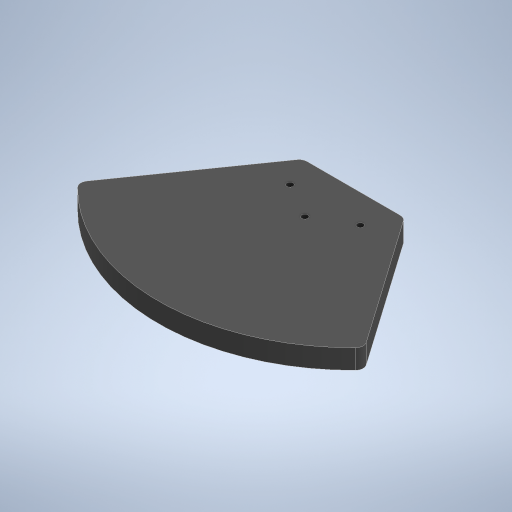
# Autodesk Inventor part: toe_sole_front
Saved by Autodesk Inventor 2024.1 (Build 281209000, 209)
## iProperties
Created: 2024-02-12
Part Number: toe_sole_front
Material: 一般
Document SubType Name: Modeling
Designer: hibik
Density: 1 g/cm^3
Appearance: 既定
Author: hibik
Autodesk Inventor part; units mm, degrees
ref_plane "YZ Plane" through (0, 0, 0) normal (1, 0, 0) x (0, 1, 0)
ref_plane "XZ Plane" through (0, 0, 0) normal (0, 1, 0) x (-1, 0, 0)
ref_plane "XY Plane" through (0, 0, 0) normal (0, 0, 1) x (1, 0, 0)
sketch "スケッチ1" plane through (0, 0, 0) normal (0, 1, 0) x (-1, 0, 0)
  line L0 (26, 0) -> (0, 0)
  line L1 (0, 0) -> (0, -15)
  line L2 (0, -15) -> (26, -15)
  line L3 (26, -15) -> (26, 0)
  line L4 (49.744, 13.9099) -> (26, -20)
  line L5 (26, -20) -> (0, -20)
  line L6 (0, -20) -> (-23.744, 13.9099)
  arc A0 (49.744, 13.9099) -> (-23.744, 13.9099) centre (13, -20) ccw
  line L7 (0, 0) -> (26, -15)
  line L8 (0, -15) -> (26, 0)
  line L9 (4, -2.3077) -> (22, -2.3077)
  line L10 (22, -2.3077) -> (22, -12.6923)
  line L11 (22, -12.6923) -> (4, -12.6923)
  line L12 (4, -12.6923) -> (4, -2.3077)
  circle A1 centre (4, -2.3077) radius 0.8
  circle A2 centre (4, -12.6923) radius 0.8
  circle A3 centre (22, -2.3077) radius 0.8
  circle A4 centre (22, -12.6923) radius 0.8
  circle A5 centre (13, -7.5) radius 0.8
  point P0 (22.6929, -13.0921)
  point P1 (21.2, -12.6923)
  dimension "d0" = 26
  dimension "d1" = 15
  dimension "d4" = 35
  dimension "d5" = 35
  dimension "d6" = 5
  dimension "d7" = 50
  dimension "d23" = 4
  dimension "d24" = 1.6
  dimension "d25" = 1.6
  dimension "d26" = 1.6
  dimension "d27" = 1.6
  dimension "d32" = 1.6
  constraints: 26 end point, 6 centre point, 6 coincident, 5 point on line, 4 parallel, 3 horizontal, 2 midpoint, 2 perpendicular, 2 point on circle
  measures "d0" distance of L0.start L0.end
  measures "d1" distance of L2.end L0.start
  measures "d4" angle of L3 L4
  measures "d5" angle of L6 L1
  measures "d6" distance between parallel lines of L5 L2
  measures "d7" radius of A0
  measures "d23" distance between parallel lines of L1 L12
  measures "d24" diameter of A1
  measures "d25" diameter of A2
  measures "d26" diameter of A3
  measures "d27" diameter of A4
  measures "d32" diameter of A5
extrude "押し出し1" add sketch "スケッチ1" along normal blind 4 contours L8 A3 L9 A1 L7 L0 | L3 L7 A4 L10 A3 L8 | L7 A1 L12 A2 L8 L1 | L2 L8 A2 L11 A4 L7 | A3 L10 L8 | L8 L9 A3 | A1 L9 L7 | L7 L12 A1 | L10 A3 L8 | L8 A3 L9 | A3 L8 A5 L7 A1 L9 | L9 A1 L7 | L7 A1 L12 | A1 L7 A5 L8 A2 L12 | L11 A2 L8 A5 L7 A4 | A3 L10 A4 L7 A5 L8 | L4 L5 L6 A0
sketch "スケッチ2" plane through (0, 0, 0) normal (0, -1, 0) x (1, 0, 0)
  arc A0 (-43.4411, 17.1126) -> (-47.1659, 13.7149) centre (-13, -20) ccw
  arc A1 (23.744, 13.9099) -> (-49.744, 13.9099) centre (-13, -20) ccw projected
  arc A2 (21.1659, 13.7149) -> (17.4411, 17.1126) centre (-13, -20) ccw
  line L0 (21.1659, 13.7149) -> (-1.0411, -18)
  line L1 (-43.4411, 17.1126) -> (-18.855, -18)
  line L2 (-47.1659, 13.7149) -> (-24.9589, -18)
  line L3 (23.744, 13.9099) -> (0, -20) projected
  line L4 (-26, -20) -> (-49.744, 13.9099) projected
  line L5 (17.4411, 17.1126) -> (-7.145, -18)
  line L6 (-24.9589, -18) -> (-18.855, -18)
  line L7 (0, -20) -> (-26, -20) projected
  line L8 (-7.145, -18) -> (-1.0411, -18)
  circle A3 centre (-4, -12.6923) radius 0.8 projected
  circle A4 centre (-22, -12.6923) radius 0.8 projected
  circle A5 centre (-4, -12.6923) radius 2.5
  circle A6 centre (-22, -12.6923) radius 2.5
  circle A7 centre (-13, -7.5) radius 0.8 projected
  circle A8 centre (-13, -7.5) radius 2.5
  arc A9 (-36.8542, 21.6531) -> (-43.4411, 17.1126) centre (-13, -20) ccw
  arc A10 (17.4411, 17.1126) -> (10.8542, 21.6531) centre (-13, -20) ccw
  line L9 (-36.8542, 21.6531) -> (-31.2525, 13.6531)
  line L10 (-31.2525, 13.6531) -> (-37.8057, 9.0645)
  line L11 (10.8542, 21.6531) -> (5.2525, 13.6531)
  line L12 (5.2525, 13.6531) -> (11.8057, 9.0645)
  point P0 (-23.792, -10.9492)
  point P1 (-20.9749, -14.9725)
  point P2 (-5.0251, -14.9725)
  point P3 (-2.208, -10.9492)
  dimension "d10" = 2
  dimension "d11" = 2
  dimension "d14" = 2
  dimension "d15" = 2
  dimension "d16" = 5
  dimension "d17" = 2
  dimension "d18" = 2
  dimension "d19" = 5
  dimension "d29" = 5
  dimension "d30" = 5
  dimension "d33" = 5
  dimension "d50" = 8
  dimension "d51" = 8
  dimension "d52" = 8
  dimension "d53" = 8
  constraints: 20 end point, 8 point on circle, 7 centre point, 6 concentric, 6 parallel, 4 perpendicular, 3 coincident, 2 point on line
  measures "d10" distance between parallel lines of L3 L0
  measures "d11" radial gap between concentric circles of A1 A2
  measures "d14" distance between parallel lines of L4 L2
  measures "d15" radial gap between concentric circles of A1 A0
  measures "d16" distance between parallel lines of L2 L1
  measures "d17" distance between parallel lines of L7 L6
  measures "d18" distance between parallel lines of L7 L8
  measures "d19" distance between parallel lines of L0 L5
  measures "d29" diameter of A5
  measures "d30" diameter of A6
  measures "d33" diameter of A8
  measures "d50" distance between parallel lines of L1 L9
  measures "d51" distance between parallel lines of L5 L11
  measures "d52" vertical distance of L11.start L11.end
  measures "d53" vertical distance of L9.start L9.end
extrude "押し出し2" add sketch "スケッチ2" along normal blind 1 contours L3 L7 L4 A1
fillet "フィレット1" radius 0.5 14 edges at (10.0624, -1, -2.1426) (16.2803, -1, 18.035) (-6.0851, -1, -16.4862) (4.7989, -1, -0.9423) (-4.0931, -1, -18) (-19.9149, -1, -16.4862) (-30.7989, -1, -0.9423) (-21.9069, -1, -18) (-36.0624, -1, -2.1426) (-42.2803, -1, 18.035) (8.0533, -1, 17.6531) (8.5291, -1, 11.3588) (-34.0533, -1, 17.6531) (-34.5291, -1, 11.3588)
extrude "押し出し3" cut sketch "スケッチ2" against normal blind 1 contours A6 L1 A4 | L1 A4 A6 | A4 L1 | L1 A4 | A5 L5 A3 | L5 A3 A5 | A3 L5 | L5 A3 | A8
fillet "フィレット2" radius 2 4 edges at (23.744, 1.5, 13.9099) (0, 1.5, -20) (-26, 1.5, -20) (-49.744, 1.5, 13.9099)
equation "\"d5\" = d4"
